Autodesk Inventor part; units mm, degrees
(part 2 of 2)
sketch "Sketch120" plane through (0, 0, 52) normal (0, 0, -1) x (-1, 0, 0)
  line L0 (-5.5, 48.7965) -> (-5.5, 49.7965) projected
  line L1 (-5.5, 47.9965) -> (-5.5, 48.7965) projected
  line L2 (-5.5, 47.9965) -> (-5.5, 45.9965) projected
  line L3 (-5.5, 45.9965) -> (-5.5, 19.7965) projected
  line L4 (-5.5, 19.7965) -> (-5.5, 45.9965) projected
  line L5 (-5.5, 45.9965) -> (-5.5, 47.9965) projected
  line L6 (-5.5, 48.7965) -> (-5.5, 47.9965) projected
  line L7 (-5.5, 49.7965) -> (-5.5, 48.7965) projected
  line L8 (-5.5, -48.7965) -> (-5.5, -49.7965) projected
  line L9 (-5.5, -47.9965) -> (-5.5, -48.7965) projected
  line L10 (-5.5, -47.9965) -> (-5.5, -45.9965) projected
  line L11 (-5.5, -45.9965) -> (-5.5, -19.7965) projected
  line L12 (-5.5, -19.7965) -> (-5.5, -45.9965) projected
  line L13 (-5.5, -45.9965) -> (-5.5, -47.9965) projected
  line L14 (-5.5, -48.7965) -> (-5.5, -47.9965) projected
  line L15 (-5.5, -49.7965) -> (-5.5, -48.7965) projected
  line L16 (-6, 5.3855) -> (-6, 46.7965) projected
  line L17 (-6, -46.7965) -> (-6, -5.3855) projected
  line L18 (-6, 46.7965) -> (-3.5, 46.7965)
  line L19 (-3.5, 46.7965) -> (-3.5, 17.7965)
  line L20 (-3.5, 17.7965) -> (-6, 17.7965)
  line L21 (-6, 17.7965) -> (-6, 46.7965)
  line L22 (-6, -46.7965) -> (-3.5, -46.7965)
  line L23 (-3.5, -46.7965) -> (-3.5, -17.7965)
  line L24 (-3.5, -17.7965) -> (-6, -17.7965)
  line L25 (-6, -17.7965) -> (-6, -46.7965)
  point P0 (0, 0)
  dimension "d491" = 2
  dimension "d492" = 2
  dimension "d493" = 2
  constraints: 16 end point, 4 parallel, 2 horizontal, 2 perpendicular, 1 vertical alignment
  measures "d491" distance between parallel lines of L19 L3
  measures "d492" distance from line of L20 L3.end
  measures "d493" distance from line of L24 L11.end
extrude "Extrusion103" add sketch "Sketch120" along normal blind 2
body "Solid2"
